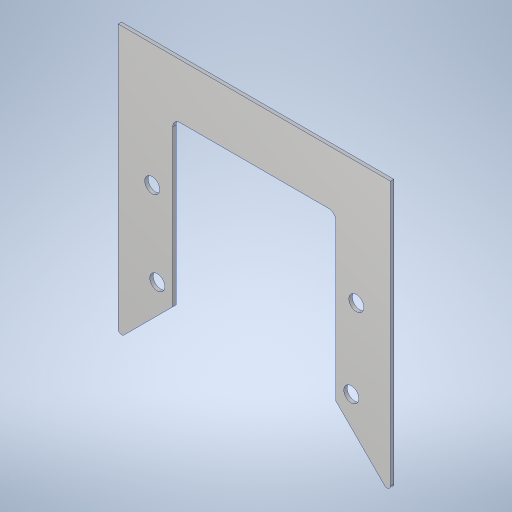
# Autodesk Inventor part: AI1-001
Saved by Autodesk Inventor 2023.4 (Build 274418000, 418)
## iProperties
Created: 2025-01-15
Part Number: AI1-001
Material: Aluminum 6061
Document SubType Name: Modeling
Designer: mavericks
Density: 2.7 g/cm^3
Appearance: Aluminum - Flat
Author: mavericks
Autodesk Inventor part; units mm, degrees
ref_plane "YZ Plane" through (0, 0, 0) normal (1, 0, 0) x (0, 1, 0)
ref_plane "XZ Plane" through (0, 0, 0) normal (0, 1, 0) x (-1, 0, 0)
ref_plane "XY Plane" through (0, 0, 0) normal (0, 0, 1) x (1, 0, 0)
sketch "Sketch1" plane through (0, 0, 0) normal (0, 0, 1) x (1, 0, 0)
  line L0 (-254, 254) -> (254, 254)
  line L1 (254, 254) -> (254, -254)
  line L2 (-254, -254) -> (-254, 254)
  line L3 (-254, 254) -> (254, -254) construction
  line L4 (254, 254) -> (-254, -254) construction
  line L5 (-254, -254) -> (-152.4, -152.4)
  line L6 (-152.4, -152.4) -> (-152.4, 152.4)
  line L7 (-152.4, 152.4) -> (152.4, 152.4)
  line L8 (152.4, 152.4) -> (152.4, -152.4)
  line L9 (254, -254) -> (152.4, -152.4)
  point P0 (0, 0)
  dimension "d2" = 101.6
  dimension "d3" = 101.6
  dimension "d23" = 304.8
  constraints: 20 end point, 4 point on line, 3 perpendicular, 2 midpoint, 1 collinear, 1 horizontal, 1 parallel, 1 vertical
  measures "d2" distance between parallel lines of L6 L2
  measures "d3" distance between parallel lines of L0 L7
  measures "d23" distance between parallel lines of L8 L6
extrude "Extrusion1" add sketch "Sketch1" along normal blind 6.35
sketch "Sketch2" plane through (0, 0, 6.35) normal (0, 0, 1) x (1, 0, 0)
  line L0 (-152.4, -152.4) -> (-152.4, 152.4) projected
  line L1 (152.4, 152.4) -> (152.4, -152.4) projected
  circle A0 centre (-180.975, -127) radius 50.8 construction
  line L2 (-254, -254) -> (-152.4, -152.4) construction
  point P0 (0, 0)
  point P1 (-190.5, 25.2039)
  point P2 (190.5, 25.2039)
  point P3 (180.975, -127)
  dimension "d6" = 28.575
  dimension "d7" = 38.1
  dimension "d8" = 38.1
  dimension "d9" = 28.575
  dimension "d18" = 152.5016
  dimension "d20" = 152.5016
  dimension "d21" = 101.6
  dimension "d25" = 127
  constraints: 1 centre point, 1 coincident, 1 horizontal alignment
  measures "d6" distance from line of L0 point (-180.975, -127)
  measures "d7" distance from line of L0 point (-190.5, 25.204)
  measures "d8" distance from line of L1 point (190.5, 25.204)
  measures "d9" distance from line of L1 point (180.975, -127)
  measures "d18" distance of point (-180.975, -127) point (-190.5, 25.204)
  measures "d20" distance of point (190.5, 25.204) point (180.975, -127)
  measures "d21" diameter of A0
  measures "d25" vertical distance of point (-180.975, -127) L2.start
hole "Hole1" at (-180.975, -127, 6.35) at (-190.5, 25.2039, 6.35) at (190.5, 25.2039, 6.35) at (180.975, -127, 6.35) direction (0, 0, -1) diameter 27.94 end through all
fillet "Fillet1" radius 13.97 2 edges at (-152.4, 152.4, 3.175) (152.4, 152.4, 3.175)
fillet "Fillet2" radius 6.35 2 edges at (-254, -254, 3.175) (254, -254, 3.175)
equation "\"d8\" = d7"
equation "\"d9\" = d6"
equation "\"d20\" = d18"
body "Solid1"
